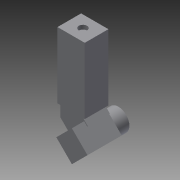
# Autodesk Inventor part: Sholder_Yaw
Saved by Autodesk Inventor 2013 (Build 170138000, 138)
## iProperties
Created: 2012-12-04
Part Number: Sholder_Yaw
Material: Generic
Document SubType Name: Modeling
Designer: Joe
Density: 1 g/cm^3
Author: Joe
Autodesk Inventor part; units mm, degrees
ref_plane "YZ Plane" through (0, 0, 0) normal (1, 0, 0) x (0, 1, 0)
ref_plane "XZ Plane" through (0, 0, 0) normal (0, 1, 0) x (-1, 0, 0)
ref_plane "XY Plane" through (0, 0, 0) normal (0, 0, 1) x (1, 0, 0)
sketch "Sketch1" plane through (0, 0, 0) normal (0, 0, 1) x (1, 0, 0)
  line L0 (0, 0) -> (29, 0)
  line L1 (29, 0) -> (29, -162)
  line L2 (29, -162) -> (0, -162)
  line L3 (0, -162) -> (0, 0) construction
  line L4 (0, 0) -> (-29, 0)
  line L5 (-29, 0) -> (-29, -162)
  line L6 (-29, -162) -> (0, -162)
  dimension "d0" = 29
  dimension "d1" = 162
  constraints: 14 end point, 2 parallel, 2 symmetric about line, 1 horizontal, 1 perpendicular
  measures "d0" distance of L0.start L0.end
  measures "d1" distance of L0.end L1.end
extrude "Extrusion1" add sketch "Sketch1" along normal mid plane 67
sketch "Sketch3" plane through (0, 0, 0) normal (1, 0, 0) x (0, 1, 0)
  line L0 (-162, 28.5) -> (-165, 28.5)
  line L1 (-165, 28.5) -> (-175.6066, 39.1066)
  line L2 (-162, 33.5) -> (0, 33.5) projected
  line L3 (-162, 33.5) -> (-162, -33.5) projected
  line L4 (-162, -28.5) -> (-190.0244, -28.5)
  line L5 (-190.0244, -28.5) -> (-216.6188, -1.9056)
  line L6 (-177.0208, 37.6924) -> (-169.2426, 29.9142)
  line L7 (-169.2426, 29.9142) -> (-207.4264, -8.2696)
  line L8 (-207.4264, -8.2696) -> (-215.2046, -0.4914)
  line L9 (-175.6066, 39.1066) -> (-177.0208, 37.6924)
  line L10 (-215.2046, -0.4914) -> (-216.6188, -1.9056)
  line L11 (0, -33.5) -> (-162, -33.5) construction
  point P0 (0, 0)
  dimension "d6" = 5
  dimension "d7" = 3
  dimension "d8" = 45
  dimension "d9" = 15
  dimension "d11" = 11
  dimension "d13" = 2
  dimension "d14" = 54
  dimension "d15" = 5
  dimension "d16" = 90
  constraints: 18 end point, 2 collinear, 2 parallel, 2 perpendicular, 2 point on line, 1 horizontal
  measures "d6" distance between parallel lines of L2 L0
  measures "d7" distance of L0.start L0.end
  measures "d8" angle of L3 L1
  measures "d9" distance of L0.end L1.end
  measures "d11" distance of L6.start L6.end
  measures "d13" distance between parallel lines of L6 L1
  measures "d14" distance between parallel lines of L8 L6
  measures "d15" distance between parallel lines of L11 L4
  measures "d16" angle of L1 L9
extrude "Extrusion2" add sketch "Sketch3" along normal mid plane 54
sketch "Sketch5" plane through (0, 0, 0) normal (1, 0, 0) x (0, 1, 0)
  line L0 (-207.4264, 68.098) -> (-169.2426, 29.9142)
  line L1 (-169.2426, 29.9142) -> (-207.4264, -8.2696)
  line L2 (-207.4264, -8.2696) -> (-245.6102, 29.9142)
  line L3 (-245.6102, 29.9142) -> (-207.4264, 68.098)
  line L4 (-169.2426, 29.9142) -> (-207.4264, -8.2696) projected
  line L5 (-177.0208, 37.6924) -> (-169.2426, 29.9142) projected
  line L6 (-207.4264, -8.2696) -> (-215.2046, -0.4914) projected
  point P0 (0, 0)
  constraints: 8 end point, 3 collinear, 2 parallel, 2 perpendicular
extrude "Extrusion3" add sketch "Sketch5" along normal mid plane 114
sketch "Sketch6" plane through (-29, 0, 33.5) normal (0, 1, 0) x (1, 0, 0)
  circle A0 centre (29, 33.5) radius 10
  dimension "d21" = 20
  constraints: 1 centre point, 1 coincident
  measures "d21" diameter of A0
extrude "Extrusion4" cut sketch "Sketch6" against normal blind 10
sketch "Sketch7" plane through (57, 0, 0) normal (1, 0, 0) x (0, 0, -1)
  line L0 (-29.9142, -169.2426) -> (-68.098, -207.4264) projected
  line L1 (-68.098, -207.4264) -> (-29.9142, -245.6102) projected
  line L2 (-29.9142, -245.6102) -> (8.2696, -207.4264) projected
  line L3 (8.2696, -207.4264) -> (-29.9142, -169.2426) projected
  line L4 (-29.9142, -245.6102) -> (-29.9142, -169.2426) construction
  circle A0 centre (-29.9142, -207.4264) radius 27
  point P0 (0, 0)
  constraints: 2 end point, 1 centre point, 1 midpoint, 1 vertical
extrude "Extrusion5" cut sketch "Sketch7" against normal blind 30 contours L3 A0 L0 | A0 L1 L0 | L3 L2 A0 | A0 L2 L1
move or copy body "Move Body1" bodies to move or copy 1 copy no rotation origin (0, 0, 0) rotation axis (1, 0, 0) rotation angle 90
move or copy body "Move Body2" bodies to move or copy 1 copy no rotation origin (0, 0, 0) rotation axis (0, 0, 1) rotation angle 90
move or copy body "Move Body3" bodies to move or copy 1 copy no translate (0, 0, -39)
body "Solid1"
